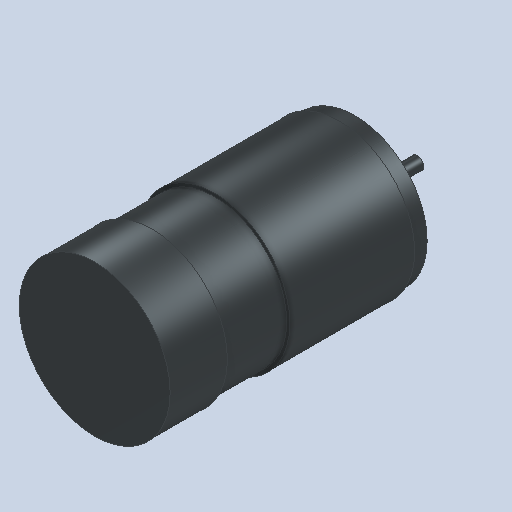
# Autodesk Inventor part: RD008_モータ(DMN29)
Saved by Autodesk Inventor 2022 (Build 260153000, 153)
## iProperties
Created: 2021-10-16
Part Number: RD008_モータ(DMN29)
Material: 鉄、鋳鉄
Document SubType Name: Modeling
Designer: gilte
Density: 7.15 g/cm^3
Appearance: 鉄 ねずみ鋳鉄
Author: gilte
Autodesk Inventor part; units mm, degrees
ref_plane "YZ Plane" through (0, 0, 0) normal (1, 0, 0) x (0, 1, 0)
ref_plane "XZ Plane" through (0, 0, 0) normal (0, 1, 0) x (-1, 0, 0)
ref_plane "XY Plane" through (0, 0, 0) normal (0, 0, 1) x (1, 0, 0)
sketch "スケッチ1" plane through (0, 0, 0) normal (0, 0, 1) x (1, 0, 0)
  circle A0 centre (0, 0) radius 1.25
  dimension "d0" = 2.5
  constraints: 1 centre point, 1 coincident
  measures "d0" diameter of A0
extrude "押し出し1" add sketch "スケッチ1" along normal blind 9.3
sketch "スケッチ2" plane through (0, 0, 9.3) normal (0, 0, 1) x (1, 0, 0)
  circle A0 centre (0, 0) radius 5
  dimension "d3" = 10
  constraints: 1 centre point, 1 coincident
  measures "d3" diameter of A0
extrude "押し出し2" add sketch "スケッチ2" along normal blind 2.7
sketch "スケッチ3" plane through (0, 0, 12) normal (0, 0, 1) x (1, 0, 0)
  circle A0 centre (0, 0) radius 5 projected
  circle A1 centre (0, 0) radius 13.9
  dimension "d6" = 27.8
  constraints: 1 centre point, 1 coincident
  measures "d6" diameter of A1
extrude "押し出し3" add sketch "スケッチ3" along normal blind 3 contours A0 | A1
sketch "スケッチ4" plane through (0, 0, 15) normal (0, 0, 1) x (1, 0, 0)
  circle A0 centre (0, 0) radius 1.25 projected
  circle A1 centre (0, 0) radius 14.5
  dimension "d9" = 29
  constraints: 1 centre point, 1 coincident
  measures "d9" diameter of A1
extrude "押し出し4" add sketch "スケッチ4" along normal blind 24 contours A0 | A1
sketch "スケッチ5" plane through (0, 0, 39) normal (0, 0, 1) x (1, 0, 0)
  circle A0 centre (0, 0) radius 13.9
  dimension "d12" = 27.8
  constraints: 1 centre point, 1 coincident
  measures "d12" diameter of A0
extrude "押し出し5" add sketch "スケッチ5" along normal blind 12
sketch "スケッチ6" plane through (0, 0, 51) normal (0, 0, 1) x (1, 0, 0)
  circle A0 centre (0, 0) radius 14.5
  dimension "d15" = 29
  constraints: 1 centre point, 1 coincident
  measures "d15" diameter of A0
extrude "押し出し6" add sketch "スケッチ6" along normal blind 11
sketch "スケッチ7" plane through (0, 0, 12) normal (0, 0, -1) x (-1, 0, 0)
  point P0 (0, 0)
  point P1 (0, -8)
  point P2 (0, 8)
  dimension "d18" = 16
  dimension "d19" = 8
  measures "d18" distance of point (0, 8) point (0, -8)
  measures "d19" distance of point (0, -8) point (0, 0)
hole "穴1" at (0, -8, 12) at (0, 8, 12) direction (0, 0, 1) diameter 2.1129 depth 3 tip angle 118 thread size "M2.6x0.45" class "6H" standard "ANSI Metric M Profile"
sketch "スケッチ8" plane through (0, 0, 12) normal (0, 0, -1) x (-1, 0, 0)
  circle A0 centre (10, 0) radius 1.25
  point P0 (0, 0)
  dimension "d27" = 2.5
  dimension "d28" = 10
  constraints: 1 centre point
  measures "d27" diameter of A0
  measures "d28" distance of point (0, 0) A0.centre
extrude "押し出し7" cut sketch "スケッチ8" against normal blind 3
equation "\"d19\" = 0.5 * d18"
